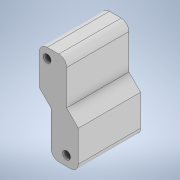
# Autodesk Inventor part: bridge_structure_C
Saved by Autodesk Inventor 2021 (Build 250183000, 183)
## iProperties
Created: 2026-02-15
Part Number: bridge_structure_C
Material: Generic
Document SubType Name: Modeling
Designer: Toby
Density: 1 g/cm^3
Appearance: Default
Author: Toby
Autodesk Inventor part; units mm, degrees
ref_plane "YZ Plane" through (0, 0, 0) normal (1, 0, 0) x (0, 1, 0)
ref_plane "XZ Plane" through (0, 0, 0) normal (0, 1, 0) x (-1, 0, 0)
ref_plane "XY Plane" through (0, 0, 0) normal (0, 0, 1) x (1, 0, 0)
sketch "Sketch1" plane through (0, 0, 0) normal (0, 0, 1) x (1, 0, 0)
  line L0 (-5, 12) -> (5, 12)
  line L1 (5, 12) -> (5, -12)
  line L2 (5, -12) -> (-5, -12)
  line L3 (-5, -12) -> (-5, 12)
  point P0 (0, 0)
  dimension "d0" = 10
  dimension "d1" = 24
  dimension "d2" = 12
  dimension "d3" = 5
  constraints: 8 end point, 2 parallel, 1 horizontal, 1 perpendicular
  measures "d0" distance of L0.start L0.end
  measures "d1" distance of L2.end L0.start
  measures "d2" distance from line of point (0, 0) L0
  measures "d3" distance from line of point (0, 0) L3
extrude "Extrusion1" add sketch "Sketch1" along normal blind 16
sketch "Sketch2" plane through (0, 0, 16) normal (0, 0, 1) x (1, 0, 0)
  line L0 (-5, -12) -> (5, -12) projected
  line L1 (5, -12) -> (5, 12) projected
  circle A0 centre (2, -9.5) radius 1
  point P0 (0, 0)
  point P1 (-2.9408, 9.031)
  dimension "d6" = 2.5
  dimension "d7" = 3
  dimension "d8" = 2
  constraints: 1 centre point, 1 coincident
  measures "d6" distance from line of L0 point (2, -9.5)
  measures "d7" distance from line of L1 point (2, -9.5)
  measures "d8" diameter of A0
extrude "Extrusion2" cut sketch "Sketch2" against normal blind 16
sketch "Sketch3" plane through (0, 0, 16) normal (0, 0, 1) x (1, 0, 0)
  circle A0 centre (2, -9.5) radius 1 projected
  circle A1 centre (-3, 9.5) radius 1
  point P0 (0, 0)
  point P1 (23.854, -2.3999)
  dimension "d11" = 5
  dimension "d12" = 19
  dimension "d13" = 2
  constraints: 1 centre point, 1 coincident
  measures "d11" horizontal distance of A0.centre point (-3, 9.5)
  measures "d12" vertical distance of A0.centre point (-3, 9.5)
  measures "d13" diameter of A1
extrude "Extrusion3" cut sketch "Sketch3" against normal blind 16 contours A1
sketch "Sketch4" plane through (0, 0, 16) normal (0, 0, 1) x (1, 0, 0)
  line L0 (-5, 12) -> (-5, -12) projected
  line L1 (-5, -12) -> (-2, -12)
  line L2 (-2, -12) -> (-2, 2)
  line L3 (-2, 2) -> (-5, 2)
  line L4 (-5, 2) -> (-5, -12)
  line L5 (5, -12) -> (5, 12) projected
  line L6 (5, 12) -> (2, 12)
  line L7 (2, 12) -> (2, -2)
  line L8 (2, -2) -> (5, -2)
  line L9 (5, -2) -> (5, 12)
  point P0 (0, 0)
  dimension "d16" = 3
  dimension "d17" = 3
  dimension "d18" = 14
  dimension "d19" = 14
  constraints: 16 end point, 4 parallel, 2 horizontal, 2 perpendicular
  measures "d16" distance between parallel lines of L0 L2
  measures "d17" distance between parallel lines of L5 L7
  measures "d18" distance between parallel lines of L6 L8
  measures "d19" distance between parallel lines of L1 L3
extrude "Extrusion4" cut sketch "Sketch4" against normal blind 16
chamfer "Chamfer1" distance 3 angle 45 2 edges at (-2, 2, 8) (2, -2, 8)
fillet "Fillet1" radius 2 4 edges at (-5, 12, 8) (2, 12, 8) (5, -12, 8) (-2, -12, 8)
body "Solid1"
